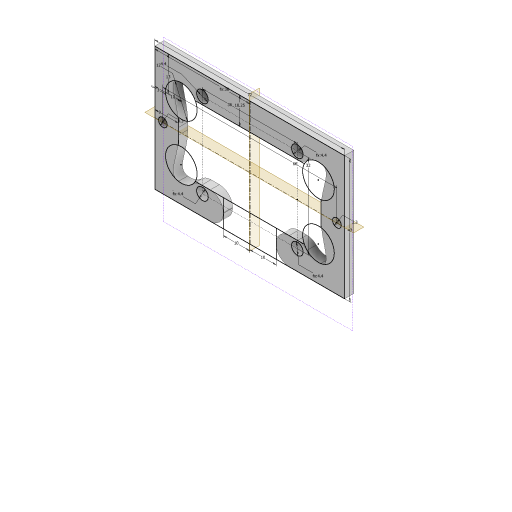
# Autodesk Inventor part: lidar_mount_frame_lidar_lite_v3hp
Saved by Autodesk Inventor 2023 (Build 270158000, 158)
## iProperties
Created: 2023-02-23
Part Number: lidar_mount_frame_lidar_lite_v3hp
Material: Generic
Document SubType Name: Modeling
Designer: Thomas
Density: 1 g/cm^3
Appearance: Default
Author: Thomas
Autodesk Inventor part; units mm, degrees
ref_plane "XY Plane" through (0, 0, 0) normal (0, 0, 1) x (1, 0, 0)
sketch "Sketch1" plane through (0, 0, 0) normal (0, 0, 1) x (1, 0, 0)
  line L0 (0, 0) -> (72, 0)
  line L1 (72, 0) -> (72, 47)
  line L2 (72, 47) -> (0, 47)
  line L3 (0, 47) -> (0, 0)
  circle A0 centre (3, 23.5) radius 1.65
  circle A1 centre (69, 23.5) radius 1.65
  line L4 (0, 23.5) -> (72, 23.5) construction
  circle A2 centre (18, 39.5) radius 2.2
  circle A3 centre (54, 39.5) radius 2.2
  circle A4 centre (54, 7.5) radius 2.2
  circle A5 centre (18, 7.5) radius 2.2
  line L5 (18, 39.5) -> (18, 7.5) construction
  line L6 (18, 7.5) -> (54, 7.5) construction
  line L7 (54, 7.5) -> (54, 39.5) construction
  line L8 (54, 39.5) -> (18, 39.5) construction
  line L9 (3.1536, 51.5748) -> (75.0735, 51.5748) construction
  line L10 (75.0735, 51.5748) -> (75.0735, -9.0389) construction
  line L11 (75.0735, -9.0389) -> (3.1536, -9.0389) construction
  line L12 (3.1536, -9.0389) -> (3.1536, 51.5748) construction
  circle A6 centre (10, 34) radius 6
  line L13 (36, 0) -> (36, 47)
  line L14 (9, 28.0839) -> (9, 23.5)
  line L15 (15.3327, 36.75) -> (36, 36.75)
  circle A7 centre (62, 34) radius 6
  line L16 (63, 28.0839) -> (63, 23.5)
  line L17 (56.6673, 36.75) -> (36, 36.75)
  circle A8 centre (10, 13) radius 6
  line L18 (9, 18.9161) -> (9, 23.5)
  line L19 (15.3327, 10.25) -> (36, 10.25)
  circle A9 centre (62, 13) radius 6
  line L20 (56.6673, 10.25) -> (36, 10.25)
  line L21 (63, 18.9161) -> (63, 23.5)
  line L22 (26, 10.25) -> (46, 10.25)
  line L23 (46, 10.25) -> (46, 0)
  line L24 (46, 0) -> (26, 0)
  line L25 (26, 0) -> (26, 10.25)
  point P0 (36, 39.5)
  point P1 (54, 23.5)
  dimension "d0" = 72
  dimension "d1" = 47
  dimension "d2" = 3.3
  dimension "d3" = 3.3
  dimension "d4" = 66
  dimension "d5" = 3
  dimension "d6" = 36
  dimension "d7" = 32
  dimension "d8" = 36
  dimension "d9" = 4.4
  dimension "d10" = 4.4
  dimension "d11" = 4.4
  dimension "d12" = 4.4
  dimension "d32" = 12
  dimension "d33" = 10
  dimension "d34" = 13
  dimension "d35" = 9
  dimension "d36" = 10.25
  dimension "d44" = 10
  dimension "d45" = 10
  constraints: 44 end point, 11 symmetric about line, 10 centre point, 8 point on circle, 7 perpendicular, 7 point on line, 6 midpoint, 4 parallel, 2 horizontal, 1 vertical, 5 other
  measures "d0" distance of L2.end L1.end
  measures "d1" distance of L1.end L0.end
  measures "d2" diameter of A0
  measures "d3" diameter of A1
  measures "d4" distance of A1.centre A0.centre
  measures "d5" distance of L4.start A0.centre
  measures "d6" distance of L7.end L5.start
  measures "d7" distance of L6.end L7.end
  measures "d8" distance from line of L3 point (36, 39.5)
  measures "d9" diameter of A2
  measures "d10" diameter of A3
  measures "d11" diameter of A5
  measures "d12" diameter of A4
  measures "d32" diameter of A6
  measures "d33" distance from line of A6.centre L3
  measures "d34" distance from line of A6.centre L2
  measures "d35" distance between parallel lines of L3 L14
  measures "d36" distance between parallel lines of L15 L2
  measures "d44" distance from line of L13.start L25
  measures "d45" distance from line of L23 L13.start
extrude "Extrusion1" add sketch "Sketch1" against normal blind 3.5 contours L3 L2 L13 L15 A6 L14 L18 A8 L19 L25 L0 | L25 L19 L13 L0 | L13 L20 L23 L0 | L2 L1 L0 L23 L20 A9 L21 L16 A7 L17 L13 | A2 | A3 | A4 | A5
extrude "Extrusion2" cut sketch "Sketch1" against normal through all draft -7 contours A2 | A3 | A4 | A5
fillet "Fillet1" radius 5 8 edges at (9, 18.9161, -1.75) (9, 28.0839, -1.75) (15.3327, 36.75, -1.75) (56.6673, 36.75, -1.75) (63, 18.9161, -1.75) (56.6673, 10.25, -1.75) (15.3327, 10.25, -1.75) (63, 28.0839, -1.75)
extrude "Extrusion3" cut sketch "Sketch1" against normal through all contours L25 L19 L13 L0 | L13 L20 L23 L0
fillet "Fillet2" radius 5 4 edges at (26, 10.25, -1.75) (46, 10.25, -1.75) (26, 0, -1.75) (46, 0, -1.75)
sketch "Sketch2" plane through (0, 0, 0) normal (0, 0, 1) x (1, 0, 0)
  arc A0 (6.7273, 18.0288) -> (9, 22.2195) centre (4, 22.2195) ccw projected
  arc A1 (6.7273, 18.0288) -> (14.258, 8.7727) centre (10, 13) ccw projected
  line L0 (9, 22.2195) -> (9, 24.7805) projected
  arc A2 (6.7273, 18.0288) -> (9, 22.2195) centre (4, 22.2195) ccw projected
  line L1 (9, 22.2195) -> (9, 14.4433) construction
  line L2 (9, 14.4433) -> (4.4748, 7.8488) construction
  arc A3 (6.7273, 18.0288) -> (14.258, 8.7727) centre (10, 13) ccw projected
  line L3 (4.4748, 7.8488) -> (9, 7.0839) construction
  spline S0 degree 3 poles (9, 22.2195) (9, 14.4433) (4.4748, 7.8488) (9, 7.0839) knots 1 1 1 1 2 2 2 2
  point P0 (0, 0)
  point P1 (8.9999, 7.0839)
  dimension "d50" = 1
  constraints: 3 tangent, 1 point on circle, 1 vertical, 3 other
  measures "d50" horizontal distance of L3.end A1.centre
extrude "Extrusion4" add sketch "Sketch2" against normal up to surface (3.5 mm away)
ref_plane "Work Plane1" through (3, 23.5, 0) normal (0, 1, 0) x (-1, 0, 0)
mirror "Mirror1" about plane through (3, 23.5, 0) normal (0, 1, 0) of "Extrusion4"
ref_plane "Work Plane2" through (36, 10.25, 0) normal (1, 0, 0) x (0, 1, 0)
mirror "Mirror2" about plane through (36, 10.25, 0) normal (1, 0, 0) of "Extrusion4", "Mirror1"
equation "\"d8\" = 0.5 * d0"
equation "\"d10\" = d9"
equation "\"d11\" = d9"
equation "\"d12\" = d9"
body "Solid1"
